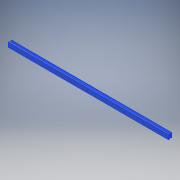
# Autodesk Inventor part: SR15W52020 Track
Saved by Autodesk Inventor 2016 (Build 200138000, 138)
## iProperties
Category: PARTsolutions
Company: THK
Created: 2015-05-03
Part Number: SR15W52020 Track
Catalog Web Link: www.cadenas.de
Description: Standard Type SR-W/T  Track-
Vendor: THK
Document SubType Name: Modeling
Designer: PARTuser1
Manufacturer: THK
Mass: 664.562 g
Surface Area: 318.483 cm^2
Volume: 85.9717 cm^3
Density: 7.73 g/cm^3
Material: Steel, Alloy
Appearance: Semi-Polished
PSOL_IDENT_0: {$CADENAS_DATA\23d-libs\thk\linear_motion_systems\lm_guide\lm_guide\lm_guide_sr\sr_wt\sr_wt_track.pr
PSOL_IDENT_1: j},201 {VTYP=3D},{NB=SR15W52020 Track},{LINA=SR15W52020 Track},{NN=Standard Type SR-W/T  Track},{DAT
PSOL_IDENT_2: E=01.03.2011 00:43:05},{GEOMDATE=28.07.2010 01:16:00},{VERSION=},{LINEID=10},{LINESUBID=-1},{WBVAR=L
PSOL_IDENT_3: ,G,GX}  {NB=SR15W52020 Track},{LINA=SR15W52020 Track},{KT=DUMMY},{MN=SR15W},{NOB=1},{L=520.0},{G=},{
PSOL_IDENT_4: GG='', 'Symmetrical (G1=G2)', 'A', 'Asymmetrical'},{GX=20},{GX1=20},{LMIN=57},{LEND=7200},{LMING=4.0
PSOL_IDENT_5: 0},{LMAXG=36.00},{M=24.00},{W=34.00},{LTR=57.00},{E=5.50},{W1=15.00},{W2=9.50},{M1=12.50},{F=60.00},
PSOL_IDENT_6: {D1=3.50},{D2=6.00},{HM=4.50},{MAXL=2500.00},{GMIN=4},{GMX=20},{GMAX1=8.533333},{G1=20},{G2=20},{NX=
PSOL_IDENT_7: 1},{H3=4.50},{LT=2400},{A=9},{LF=-10},{LM=540},{LL=1070},{AA=8},{GMAX=36},{P=9},{PX=0},{VG=8},{VGG=2
PSOL_IDENT_8: 0},{VG1=-1},{VG2=9},{ND=1.000},{GA=20.000}
SUPPLIER: THK
ARTICLENO: SR15W52020 Track
BOMINFO: SR15W52020 Track
CREATOR: CADENAS GmbH
Title: SR15W52020 Track
Author: Cadenas PARTsolutions
Autodesk Inventor part; units mm, degrees
sketch "Sketch_15" plane through (-20, 0, 0) normal (1, 0, 0) x (0, 0, -1)
  line L0 (-7.5, 0.85) -> (-6.65, 0)
  line L1 (-6.65, 0) -> (6.65, 0)
  line L2 (6.65, 0) -> (7.5, 0.85)
  line L3 (7.5, 0.85) -> (7.5, 4.768)
  line L4 (7.5, 4.768) -> (5.4163, 5.9696)
  arc A0 (5.1599, 6.9262) -> (5.4163, 5.9696) centre (5.766, 6.576) ccw
  line L5 (5.1599, 6.9262) -> (6.6573, 9.518)
  arc A1 (7.5, 10.8638) -> (6.6573, 9.518) centre (8.107, 9.547) ccw
  line L6 (7.5, 10.8638) -> (7.5, 12.05)
  line L7 (7.5, 12.05) -> (7.05, 12.5)
  line L8 (7.05, 12.5) -> (6.6661, 12.5)
  arc A2 (4.8439, 12.5) -> (6.6661, 12.5) centre (5.755, 13.628) ccw
  line L9 (4.8439, 12.5) -> (-4.8439, 12.5)
  arc A3 (-6.6661, 12.5) -> (-4.8439, 12.5) centre (-5.755, 13.628) ccw
  line L10 (-6.6661, 12.5) -> (-7.05, 12.5)
  line L11 (-7.05, 12.5) -> (-7.5, 12.05)
  line L12 (-7.5, 12.05) -> (-7.5, 10.8638)
  arc A4 (-6.6573, 9.518) -> (-7.5, 10.8638) centre (-8.107, 9.547) ccw
  line L13 (-6.6573, 9.518) -> (-5.1599, 6.9262)
  arc A5 (-5.4163, 5.9696) -> (-5.1599, 6.9262) centre (-5.766, 6.576) ccw
  line L14 (-5.4163, 5.9696) -> (-7.5, 4.768)
  line L15 (-7.5, 4.768) -> (-7.5, 0.85)
  constraints: 32 end point, 12 point on circle, 6 centre point
extrude "Extrusion1" add sketch "Sketch_15" along normal blind 520
sketch "Sketch2" plane through (-20, 12.5, -4.8439) normal (0, 1, 0) x (1, 0, 0)
  point P0 (20, -4.8439)
hole "Hole1" at (0, 12.5, 0) direction (0, -1, 0) diameter 3.5 depth 12.5 counterbore diameter 6 counterbore depth 4.5
pattern_linear "Rectangular Pattern1" count 9 spacing 60 along (1, 0, 0) of "Hole1"
ref_plane "4DUMMY_XY" through (0, 0, 0) normal (1, 0, 0) x (0, 0, -1)
ref_plane "4DUMMY_YZ" through (0, 0, 0) normal (0, 0, -1) x (0, 1, 0)
ref_plane "4DUMMY_ZX" through (0, 0, 0) normal (0, 1, 0) x (1, 0, 0)
ref_plane "4SLIDE_XY" through (-20, 4.5, 0) normal (1, 0, 0) x (0, 0, -1)
ref_plane "4SLIDE_YZ" through (-20, 4.5, 0) normal (0, 0, -1) x (0, 1, 0)
ref_plane "4SLIDE_ZX" through (-20, 4.5, 0) normal (0, 1, 0) x (1, 0, 0)
ref_plane "4TRACK_XY" through (0, 0, 0) normal (0, 0, 1) x (1, 0, 0)
ref_plane "4TRACK_YZ" through (0, 0, 0) normal (1, 0, 0) x (0, 1, 0)
ref_plane "4TRACK_ZX" through (0, 0, 0) normal (0, 1, 0) x (0, 0, 1)
body "Solid1"
